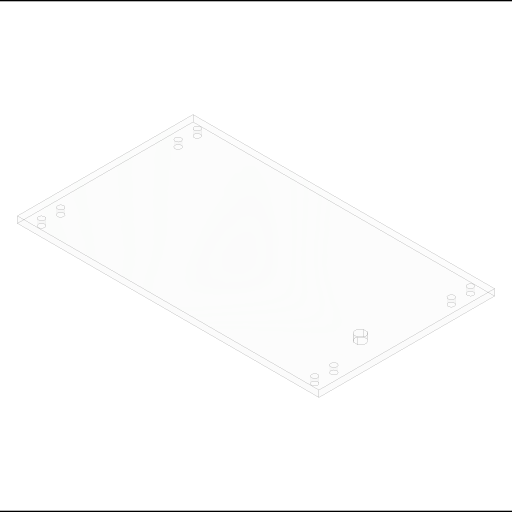
# Autodesk Inventor part: 2023 1 17 Computer Box Door
Saved by Autodesk Inventor 2023 (Build 270158000, 158)
## iProperties
Created: 2023-01-17
Part Number: 2023 1 17 Computer Box Door
Material: Polycarbonate, Clear
Document SubType Name: Modeling
Designer: kamer
Density: 1.2 g/cm^3
Appearance: Polycarbonate - Clear
Author: kamer
Autodesk Inventor part; units mm, degrees
ref_plane "YZ Plane" through (0, 0, 0) normal (1, 0, 0) x (0, 1, 0)
ref_plane "XZ Plane" through (0, 0, 0) normal (0, 1, 0) x (-1, 0, 0)
ref_plane "XY Plane" through (0, 0, 0) normal (0, 0, 1) x (1, 0, 0)
sketch "Sketch1" plane through (0, 0, 0) normal (0, 1, 0) x (-1, 0, 0)
  line L0 (0, 0) -> (-269.875, 0)
  line L1 (-269.875, 0) -> (-269.875, -157.1625)
  line L2 (-269.875, -157.1625) -> (0, -157.1625)
  line L3 (0, -157.1625) -> (0, 0)
  circle A0 centre (-257.175, -148.2725) radius 2.7559
  circle A1 centre (-257.175, -8.89) radius 2.7559
  circle A2 centre (-12.7, -8.89) radius 2.7559
  circle A3 centre (-257.175, -131.1275) radius 2.7559
  circle A4 centre (-257.175, -26.035) radius 2.7559
  circle A5 centre (-12.7, -148.2725) radius 2.7559
  circle A6 centre (-12.7, -131.1275) radius 2.7559
  circle A7 centre (-12.7, -26.035) radius 2.7559
  circle A8 centre (-244.475, -62.5475) radius 4.6609
  line L4 (-242.5434, -66.7893) -> (-246.4066, -66.7893)
  line L5 (-254, -66.7893) -> (-254, -58.3057) construction
  line L6 (-246.4066, -58.3057) -> (-242.5434, -58.3057)
  line L7 (-236.5375, -58.3057) -> (-236.5375, -66.7893) construction
  dimension "d0" = 157.1625
  dimension "d1" = 269.875
  dimension "d2" = 12.7
  dimension "d3" = 8.89
  dimension "d6" = 8.89
  dimension "d7" = 12.7
  dimension "d8" = 12.7
  dimension "d9" = 8.89
  dimension "d11" = 5.5118
  dimension "d12" = 5.5118
  dimension "d13" = 5.5118
  dimension "d15" = 17.145
  dimension "d16" = 12.7
  dimension "d17" = 5.5118
  dimension "d18" = 5.5118
  dimension "d19" = 12.7
  dimension "d20" = 17.145
  dimension "d21" = 12.7
  dimension "d22" = 8.89
  dimension "d23" = 5.5118
  dimension "d24" = 17.145
  dimension "d25" = 12.7
  dimension "d26" = 5.5118
  dimension "d27" = 12.7
  dimension "d28" = 17.145
  dimension "d29" = 5.5118
  dimension "d32" = 25.4
  dimension "d33" = 9.3218
  dimension "d34" = 4.2418
  dimension "d35" = 4.2418
  dimension "d36" = 17.4625
  dimension "d37" = 15.875
  dimension "d38" = 94.615
  constraints: 16 end point, 9 centre point, 4 parallel, 4 point on circle, 2 horizontal, 2 perpendicular
  measures "d0" distance between parallel lines of L0 L2
  measures "d1" distance of L1.end L2.end
  measures "d2" distance from line of L1 A0.centre
  measures "d3" distance from line of L2 A0.centre
  measures "d6" distance from line of L0 A1.centre
  measures "d7" distance from line of L1 A1.centre
  measures "d8" distance from line of L3 A2.centre
  measures "d9" distance from line of L0 A2.centre
  measures "d11" diameter of A0
  measures "d12" diameter of A1
  measures "d13" diameter of A2
  measures "d15" distance of A3.centre A0.centre
  measures "d16" distance from line of L1 A3.centre
  measures "d17" diameter of A3
  measures "d18" diameter of A4
  measures "d19" distance from line of L1 A4.centre
  measures "d20" distance of A1.centre A4.centre
  measures "d21" distance from line of L3 A5.centre
  measures "d22" distance from line of L2 A5.centre
  measures "d23" diameter of A5
  measures "d24" distance of A6.centre A5.centre
  measures "d25" distance from line of L3 A6.centre
  measures "d26" diameter of A6
  measures "d27" distance from line of L3 A7.centre
  measures "d28" distance of A2.centre A7.centre
  measures "d29" diameter of A7
  measures "d32" distance from line of L1 A8.centre
  measures "d33" diameter of A8
  measures "d34" distance from line of L4 A8.centre
  measures "d35" distance from line of L6 A8.centre
  measures "d36" distance between parallel lines of L7 L5
  measures "d37" distance between parallel lines of L1 L5
  measures "d38" distance from line of A8.centre L2
extrude "Extrusion2" add sketch "Sketch1" along normal blind 5.7658 contours L3 L2 L1 L0 | L6 A8 | A8 L4
body "Solid2"
